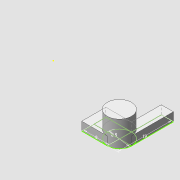
# Autodesk Inventor part: Spacer
Saved by Autodesk Inventor 2013 SP2 (Build 170200200, 200)
## iProperties
Created: 2014-04-23
Part Number: Spacer
Material: Generic
Document SubType Name: Modeling
Designer: Kevin
Density: 1 g/cm^3
Author: Kevin
Autodesk Inventor part; units mm, degrees
ref_plane "YZ Plane" through (0, 0, 0) normal (1, 0, 0) x (0, 1, 0)
ref_plane "XZ Plane" through (0, 0, 0) normal (0, 1, 0) x (-1, 0, 0)
ref_plane "XY Plane" through (0, 0, 0) normal (0, 0, 1) x (1, 0, 0)
sketch "Sketch1" plane through (0, 0, 0) normal (0, 1, 0) x (-1, 0, 0)
  arc A0 (-31.1503, 12.1688) -> (-35.4003, 7.9188) centre (-35.4003, 12.1688) ccw
  line L0 (-35.4003, 16.4188) -> (-35.4003, -2.5812)
  line L1 (-39.6503, 12.1688) -> (-31.1503, 12.1688)
  line L2 (-39.6503, -2.5812) -> (-39.6503, 12.1688)
  line L3 (-35.4003, 12.1688) -> (-26.4003, 12.1688)
  line L4 (-35.4003, 16.4188) -> (-26.4003, 16.4188)
  line L5 (-26.4003, 16.4188) -> (-26.4003, 7.9188)
  line L6 (-26.4003, 7.9188) -> (-35.4003, 7.9188)
  line L7 (-35.4003, 7.9188) -> (-35.4003, 16.4188)
  arc A1 (-35.4003, 7.9188) -> (-31.1503, 12.1688) centre (-35.4003, 12.1688) ccw
  line L8 (-35.4003, -2.5812) -> (-39.6503, -2.5812)
  point P0 (0, 0)
  dimension "d0" = 8.5
  dimension "d3" = 19
  dimension "d4" = 9
  constraints: 18 end point, 6 point on circle, 3 parallel, 2 centre point, 2 horizontal, 2 perpendicular, 1 point on line
  measures "d0" diameter of A0
  measures "d3" distance of L0.start L0.end
  measures "d4" distance of L3.start L3.end
extrude "Extrusion2" add sketch "Sketch1" along normal blind 3
extrude "Extrusion3" add sketch "Sketch1" along normal blind 7 contours L1 L0 A0 | A1 L0 L1 | L0 L1 A0 | L0 A0 L1
sketch "Sketch2" plane through (35.4003, 7, 12.1688) normal (0, 1, 0) x (1, 0, 0)
  circle A0 centre (0, 0) radius 4.25 projected
  circle A1 centre (0, 0) radius 4.25
  point P0 (-35.4003, 12.1688)
  constraints: 1 centre point, 1 coincident, 1 concentric
hole "Hole1" at (35.4003, 7, 12.1688) direction (0, -1, 0) diameter 2.4384 end through all
mirror "Mirror1" about plane through (39.6503, 0, -2.5812) normal (0, 0, -1) of "Extrusion2", "Extrusion3", "Hole1"
mirror "Mirror2" about plane through (26.4003, 0, -13.0812) normal (-1, 0, 0) of "Extrusion2", "Extrusion3", "Hole1", "Mirror1"
body "Solid2"
